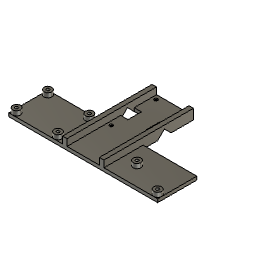
follower_arm (Autodesk Fusion 360 archive; units mm, degrees)
design "Simple Base"
Autodesk Fusion 360 part; units mm, degrees
sketch "Sketch1" plane through (0, 0, 0) normal (0, 0, 1) x (1, 0, 0) in component "Base"
  line L0 (0, 0) -> (0, 80)
  line L1 (0, 80) -> (18.5, 80)
  line L2 (18.5, 80) -> (18.5, 35)
  line L3 (18.5, 35) -> (66.5, 35)
  line L4 (66.5, 35) -> (66.5, 0)
  line L5 (66.5, 0) -> (0, 0)
  circle A0 centre (11, 76) radius 1.5
  circle A1 centre (11, 36) radius 1.5
  line L6 (14.5, 80) -> (14.5, 0)
  line L7 (18.5, 35) -> (18.5, 0)
  line L8 (8, 60) -> (8, 48)
  line L9 (8, 48) -> (14.5, 48)
  line L10 (14.5, 48) -> (14.5, 60)
  line L11 (14.5, 60) -> (8, 60)
  dimension "d1" = 80
  dimension "d4" = 3
  dimension "d5" = 11
  dimension "d8" = 0
  dimension "d9" = -40
  dimension "d10" = 4
  dimension "d17" = 14.5
  dimension "d18" = 4
  dimension "d21" = 48
  dimension "d22" = 35
  dimension "d100" = 12
  dimension "d101" = 16
  dimension "d102" = 14.5
  dimension "d103" = 8
  constraint coincident L0.start L5.end
  constraint vertical L0
  constraint perpendicular L0 L1
  constraint perpendicular L1 L2
  constraint perpendicular L0 L3
  constraint perpendicular L1 L4
  constraint perpendicular L0 L5
  constraint coincident L1 L6.start
  constraint coincident L5 L6.end
  constraint perpendicular L5 L6
  constraint coincident L5 L7.end
  constraint perpendicular L5 L7
  constraint parallel L0 L8
  constraint perpendicular L0 L9
  constraint perpendicular L9 L10
  constraint perpendicular L8 L11
  measures "d1" distance of L0.start L0.end
  measures "d4" diameter of A0
  measures "d5" distance of L0 A0.centre
  measures "d10" distance of L1 A0.centre
  measures "d17" distance of L0 L6
  measures "d18" distance of L2 L6
  measures "d21" distance of L4 L7
  measures "d22" distance of L3 L5
  measures "d100" distance of L9 L11
  measures "d101" distance of A0.centre L11
  measures "d102" distance of L0 L10
  measures "d103" distance of L0 L8
extrude "Extrude1" add sketch "Sketch1" along normal blind 3 contours L0 L1 L5 L6 L8 L9 L11 | L1 L2 L5 L6 L7 L10 | L3 L4 L5 L7 in component "Base"
extrude "Extrude2" add sketch "Sketch1" along normal blind 9 contours L1 L2 L5 L6 L7 L10 in component "Base"
chamfer "Chamfer1" distance 2 angle 45 2 edges at (9.6015, 76.5424, 0) (9.6015, 36.5424, 0) in component "Base"
sketch "Sketch7" plane through (18.5, 0, 0) normal (1, 0, 0) x (0, 1, 0) in component "Base"
  line L0 (35, 0) -> (80, 0)
  line L1 (80, 0) -> (80, 9)
  line L2 (80, 9) -> (0, 9)
  line L3 (0, 9) -> (0, 3)
  line L4 (0, 3) -> (35, 3)
  line L5 (35, 3) -> (35, 0)
  line L6 (48, 0) -> (54, 6)
  line L7 (54, 6) -> (60, 0)
  line L8 (48, 0) -> (60, 0)
  dimension "d104" = 45
  dimension "d105" = 45
  dimension "d106" = 20
  dimension "d107" = 12
  constraint coincident L0 L6.start
  constraint coincident L0 L7.end
  measures "d104" angle of L6 L8
  measures "d105" angle of L7 L8
  measures "d106" distance of L1 L7.end
  measures "d107" distance of L6.start L7.end
extrude "Extrude10" cut sketch "Sketch7" against normal blind 4 contours L0 L6 L7 L8 in component "Base"
mirror "Mirror1" about plane through (0, 0, 0) normal (1, 0, 0) of bodies 1 merged in component "Base"
sketch "Sketch2" plane through (0, 0, 3) normal (0, 0, 1) x (-1, 0, 0) in component "Base"
  line L0 (18.5, 0) -> (18.5, -35)
  line L1 (18.5, -35) -> (66.5, -35)
  line L2 (66.5, -35) -> (66.5, 0)
  line L3 (66.5, 0) -> (18.5, 0)
  circle A0 centre (63, -31.5) radius 3.5
  circle A1 centre (26, -31.5) radius 3.5
  circle A2 centre (63, -3.5) radius 3.5
  circle A3 centre (26, -3.5) radius 3.5
  circle A4 centre (63, -31.5) radius 1.35
  circle A5 centre (26, -31.5) radius 1.35
  circle A6 centre (63, -3.5) radius 1.35
  circle A7 centre (26, -3.5) radius 1.35
  dimension "d23" = 7
  dimension "d26" = -37
  dimension "d27" = 28
  dimension "d97" = 2.7
  constraint tangent L3 A2
  constraint tangent L2 A2
  constraint concentric A0 A4
  measures "d23" diameter of A0
  measures "d97" diameter of A4
extrude "Extrude3" add sketch "Sketch2" along normal blind 4 contours A1 | A3 | A2 | A0 in component "Base"
sketch "Sketch5" plane through (0, 0, 3) normal (0, 0, 1) x (-1, 0, 0) in component "Base"
  line L0 (-18.5, -35) -> (-18.5, 0)
  line L1 (-18.5, 0) -> (-66.5, 0)
  line L2 (-66.5, 0) -> (-66.5, -35)
  line L3 (-66.5, -35) -> (-18.5, -35)
  circle A0 centre (-31.5949, -16.5277) radius 3.5
  circle A1 centre (-63, -3.5) radius 3.5
  circle A2 centre (-31.5949, -16.5277) radius 1.35
  circle A3 centre (-63, -3.5) radius 1.35
  line L4 (-66.5, -35) -> (-66.5, 0)
  line L5 (-66.5, 0) -> (0, 0)
  dimension "d68" = 7
  dimension "d69" = 7
  dimension "d70" = 34
  dimension "d93" = 2.7
  dimension "d94" = 2.7
  constraint concentric A0 A2
  constraint concentric A1 A3
  constraint tangent A1 L4
  constraint tangent A1 L5
  measures "d68" diameter of A0
  measures "d69" diameter of A1
  measures "d70" distance of A0.centre A1.centre
  measures "d93" diameter of A2
  measures "d94" diameter of A3
extrude "Extrude8" add sketch "Sketch5" along normal blind 4 contours A1 | A0 in component "Base"
component "Base" placed x (1, 0, 0) y (0, 1, 0) z (0, 0, 1) at (0, 0, 0)
equation "d5 = ( 22 / 2 ) * 1 mm"
equation "d17 = ( 29 / 2 ) * 1 mm"

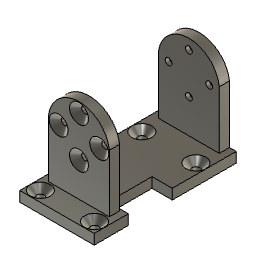
design "servo connector angle"
Autodesk Fusion 360 part; units mm, degrees
sketch "Sketch1" plane through (0, 0, 0) normal (0, 0, 1) x (1, 0, 0) in component "shoulder_rotation"
  line L0 (0, 0) -> (22, 0)
  line L1 (22, 0) -> (22, 42)
  line L2 (22, 42) -> (0, 42)
  line L3 (0, 42) -> (0, 0)
  dimension "d1" = 22
  dimension "d2" = 42
  constraint coincident L0.start L3.end
  constraint horizontal L0
  constraint perpendicular L0 L1
  constraint perpendicular L1 L2
  constraint perpendicular L0 L3
  measures "d1" distance of L0.start L0.end
  measures "d2" distance of L0.end L1.end
extrude "Extrude1" add sketch "Sketch1" along normal blind 3 in component "shoulder_rotation"
sketch "Sketch2" plane through (0, 0, 0) normal (0, 0, -1) x (1, 0, 0) in component "shoulder_rotation"
  line L0 (0, 0) -> (0, -42)
  line L1 (0, -42) -> (22, -42)
  line L2 (22, -42) -> (22, 0)
  line L3 (22, 0) -> (0, 0)
  circle A0 centre (18.9924, -33.1033) radius 1.15
  circle A1 centre (2.9924, -33.1033) radius 1.15
  circle A2 centre (18.9924, -3.1033) radius 1.15
  circle A3 centre (2.9924, -3.1033) radius 1.15
  dimension "d5" = 2.3
  dimension "d8" = -16
  dimension "d9" = 30
  measures "d5" diameter of A0
extrude "Extrude2" cut sketch "Sketch2" against normal blind 3 contours A0 | A1 | A2 | A3 in component "shoulder_rotation"
sketch "Sketch3" plane through (0, 0, 3) normal (0, 0, 1) x (-1, 0, 0) in component "shoulder_rotation"
  circle A0 centre (-2.9924, -33.1033) radius 1.15
  circle A1 centre (-2.9924, -3.1033) radius 1.15
  circle A2 centre (-18.9924, -33.1033) radius 1.15
  circle A3 centre (-18.9924, -3.1033) radius 1.15
  line L0 (0, -42) -> (0, 0)
  line L1 (0, 0) -> (-22, 0)
  line L2 (-22, 0) -> (-22, -42)
  line L3 (-22, -42) -> (0, -42)
  line L4 (-2, -42) -> (-20, -42)
  line L5 (-20, -42) -> (-20, -39)
  line L6 (-20, -39) -> (-2, -39)
  line L7 (-2, -42) -> (-2, -39)
  line L8 (-2, -9.5) -> (-20, -9.5)
  line L9 (-20, -9.5) -> (-20, -6.5)
  line L10 (-2, -9.5) -> (-2, -6.5)
  line L11 (-2, -6.5) -> (-20, -6.5)
  dimension "d14" = 29.5
  dimension "d23" = 2
  dimension "d24" = 2
  dimension "d25" = 2
  dimension "d26" = 2
  dimension "d32" = 3
  dimension "d38" = 3
  constraint perpendicular L0 L6
  constraint perpendicular L2 L8
  constraint perpendicular L8 L9
  constraint perpendicular L9 L11
  constraint vertical L10
  constraint coincident L6 L7.end
  constraint coincident L4 L7.start
  constraint coincident L6 L5.end
  constraint coincident L4 L5.start
  constraint coincident L3 L4.end
  constraint coincident L8.end L9.start
  constraint perpendicular L6 L7
  constraint coincident L4.end L5.start
  constraint coincident L5.end L6.start
  constraint perpendicular L5 L6
  measures "d14" distance of L6 L8
  measures "d23" distance of L2 L9
  measures "d24" distance of L0 L10
  measures "d25" distance of L2 L5
  measures "d26" distance of L0 L7
  measures "d32" distance of L8 L11
  measures "d38" distance of L4 L6
extrude "Extrude3" add sketch "Sketch3" along normal blind 25 contours L3 L4 L5 L6 L7 | L8 L9 L10 L11 in component "shoulder_rotation"
sketch "Sketch4" plane through (0, 42, 0) normal (0, 1, 0) x (-1, 0, 0) in component "shoulder_rotation"
  line L0 (-22, 0) -> (0, 0)
  line L1 (0, 0) -> (0, 3)
  line L2 (-2, 28) -> (-20, 28)
  line L3 (-20, 28) -> (-20, 3)
  circle A0 centre (-10.9998, 25) radius 1
  circle A1 centre (-5, 19.0002) radius 1
  circle A2 centre (-10.9998, 13.0004) radius 1
  circle A3 centre (-16.9996, 19.0002) radius 1
  line L4 (-16.9996, 19.0002) -> (-10.9998, 25) construction
  line L5 (-10.9998, 25) -> (-5, 19.0002) construction
  line L6 (-5, 19.0002) -> (-10.9998, 13.0004) construction
  line L7 (-10.9998, 13.0004) -> (-16.9996, 19.0002) construction
  line L8 (0, 3) -> (-2, 3)
  line L9 (-2, 3) -> (-2, 28)
  line L10 (-20, 3) -> (-22, 3)
  line L11 (-22, 3) -> (-22, 0)
  line L12 (-5, 19.0002) -> (-16.9996, 19.0002) construction
  arc A4 (-2, 19.9469) -> (-20, 20.0431) centre (-11.0057, 18.938) ccw
  dimension "d17" = 2
  dimension "d18" = 2
  dimension "d19" = 2
  dimension "d20" = 2
  dimension "d21" = 8.485
  dimension "d22" = 8.485
  dimension "d27" = 3
  dimension "d28" = 3
  constraint coincident A3.centre L4.start
  constraint coincident A0.centre L4.end
  constraint coincident A1.centre L5.end
  constraint coincident A2.centre L6.end
  constraint perpendicular L4 L5
  constraint perpendicular L5 L6
  constraint perpendicular L6 L7
  constraint horizontal L12
  constraint coincident L9 A4.start
  constraint coincident L3 A4.end
  measures "d17" diameter of A0
  measures "d18" diameter of A1
  measures "d19" diameter of A2
  measures "d20" diameter of A3
  measures "d21" distance of A0.centre A1.centre
  measures "d22" distance of A1.centre A2.centre
  measures "d27" distance of A1.centre L9
  measures "d28" distance of L2 A0.centre
extrude "Extrude4" cut sketch "Sketch4" against normal blind 40 contours L2 L3 A4 | L2 L9 A4 | A0 | A1 | A2 | A3 in component "shoulder_rotation"
chamfer "Chamfer1" distance 1.8 angle 45 12 edges at (17.9319, 42, 18.6386) (11.9321, 42, 24.6384) (5.9323, 42, 18.6386) (11.9321, 42, 12.6388) (17.9202, 33.5192, 3) (1.9202, 33.5192, 3) (1.9202, 3.5192, 3) (17.9202, 3.5192, 3) (17.9319, 6.5, 18.6386) (11.9321, 6.5, 24.6384) (5.9323, 6.5, 18.6386) (11.9321, 6.5, 12.6388) in component "shoulder_rotation"
sketch "Sketch5" plane through (0, 0, 0) normal (0, 0, -1) x (1, 0, 0) in component "shoulder_rotation"
  circle A0 centre (2.9924, -33.1033) radius 1.15
  circle A1 centre (2.9924, -3.1033) radius 1.15
  circle A2 centre (18.9924, -33.1033) radius 1.15
  circle A3 centre (18.9924, -3.1033) radius 1.15
  line L0 (0, 0) -> (0, -42)
  line L1 (0, -42) -> (22, -42)
  line L2 (22, -42) -> (22, 0)
  line L3 (22, 0) -> (0, 0)
  line L4 (0, -23.1033) -> (6, -23.1033)
  line L5 (6, -23.1033) -> (6, -10.1033)
  line L6 (6, -10.1033) -> (0, -10.1033)
  line L7 (11, 0) -> (11, -42) construction
  line L8 (16, -23.1033) -> (16, -10.1033)
  line L9 (16, -10.1033) -> (22, -10.1033)
  line L10 (22, -23.1033) -> (16, -23.1033)
  line L11 (11, 0) -> (11, -42) construction
  dimension "d33" = 6
  dimension "d34" = 7
  dimension "d35" = 13
  constraint coincident L0 L4.start
  constraint perpendicular L0 L4
  constraint perpendicular L4 L5
  constraint coincident L0 L6.end
  constraint perpendicular L0 L6
  constraint midpoint L3 L7.start
  constraint midpoint L1 L7.end
  constraint symmetric L4.start L7 L10.start
  constraint symmetric L4.end L7 L8.start
  constraint symmetric L5.end L7 L8.end
  constraint symmetric L6.end L7 L9.end
  constraint symmetric L11.start L7 L7.start
  constraint symmetric L11.end L7 L7.end
  measures "d33" distance of L4.start L4.end
  measures "d34" distance of A1.centre L6
  measures "d35" distance of L4 L6
extrude "Extrude5" cut sketch "Sketch5" against normal blind 3 contours L0 L4 L5 L6 | L2 L8 L9 L10 in component "shoulder_rotation"
component "shoulder_rotation" placed x (1, 0, 0) y (0, 1, 0) z (0, 0, 1) at (0, 0, 0)
